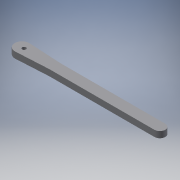
# Autodesk Inventor part: slider_link_p6
Saved by Autodesk Inventor 2017 (Build 210142000, 142)
## iProperties
Created: 2018-02-05
Part Number: slider_link_p6
Material: Generic
Document SubType Name: Modeling
Designer: Nic
Density: 1 g/cm^3
Appearance: Default
Author: Nic
Autodesk Inventor part; units mm, degrees
ref_plane "YZ Plane" through (0, 0, 0) normal (1, 0, 0) x (0, 1, 0)
ref_plane "XZ Plane" through (0, 0, 0) normal (0, 1, 0) x (-1, 0, 0)
ref_plane "XY Plane" through (0, 0, 0) normal (0, 0, 1) x (1, 0, 0)
sketch "Sketch1" plane through (0, 0, 0) normal (0, 0, 1) x (1, 0, 0)
  circle A0 centre (0, 0) radius 0.925
  line L0 (15, 2.6) -> (-0.8022, 3.4944)
  arc A1 (-0.8022, 3.4944) -> (-0.8022, -3.4944) centre (-1, 0) ccw
  line L1 (-0.8022, -3.4944) -> (15, -2.6)
  line L2 (0, 0) -> (26, 0) construction
  line L3 (15, 2.6) -> (66, 2.6)
  arc A2 (66, -2.6) -> (66, 2.6) centre (66, 0) ccw
  line L4 (66, -2.6) -> (15, -2.6)
  dimension "d0" = 1.85
  dimension "d7" = 3.5
  dimension "d8" = 1
  dimension "d10" = 2.6
  dimension "d11" = 66
  dimension "d12" = 16
  constraints: 10 end point, 4 point on circle, 4 tangent, 3 centre point, 3 horizontal, 2 horizontal alignment, 1 coincident, 1 equal length, 1 other
  measures "d0" diameter of A0
  measures "d7" radius of A1
  measures "d8" distance of A1.centre point (0, 0)
  measures "d10" radius of A2
  measures "d11" distance of point (0, 0) A2.centre
  measures "d12" horizontal distance of L0.start A1.centre
extrude "Extrusion1" add sketch "Sketch1" along normal blind 3
body "Solid1"
